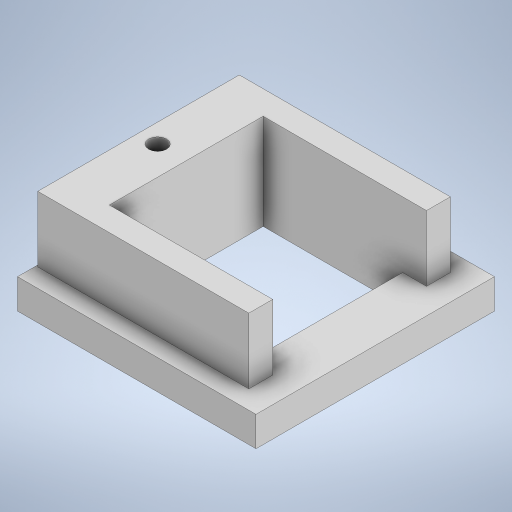
# Autodesk Inventor part: RJ45Insert
Saved by Autodesk Inventor 2024 (Build 280153000, 153)
## iProperties
Created: 2025-09-21
Part Number: RJ45Insert
Material: Generic
Document SubType Name: Modeling
Designer: Martin
Density: 1 g/cm^3
Appearance: Default
Author: Martin
Autodesk Inventor part; units mm, degrees
ref_plane "YZ Plane" through (0, 0, 0) normal (1, 0, 0) x (0, 1, 0)
ref_plane "XZ Plane" through (0, 0, 0) normal (0, 1, 0) x (-1, 0, 0)
ref_plane "XY Plane" through (0, 0, 0) normal (0, 0, 1) x (1, 0, 0)
sketch "Sketch1" plane through (0, 0, 0) normal (0, 1, 0) x (-1, 0, 0)
  line L0 (-12.7, 12.7) -> (12.7, 12.7)
  line L1 (12.7, 12.7) -> (12.7, -12.7)
  line L2 (12.7, -12.7) -> (-12.7, -12.7)
  line L3 (-12.7, -12.7) -> (-12.7, 12.7)
  line L4 (-12.7, 12.7) -> (12.7, -12.7) construction
  line L5 (12.7, 12.7) -> (-12.7, -12.7) construction
  point P0 (0, 0)
  dimension "d0" = 25.4
  dimension "d1" = 25.4
  constraints: 12 end point, 2 midpoint, 2 parallel, 1 horizontal, 1 perpendicular
  measures "d0" distance of L1.end L2.end
  measures "d1" distance of L0.end L1.end
extrude "Extrusion1" add sketch "Sketch1" along normal blind 3.175
sketch "Sketch2" plane through (0, 3.175, 0) normal (0, 1, 0) x (1, 0, 0)
  line L0 (7.4295, -8.1915) -> (-7.4295, -8.1915)
  line L1 (-7.4295, -8.1915) -> (-7.4295, 8.1915)
  line L2 (-7.4295, 8.1915) -> (7.4295, 8.1915)
  line L3 (7.4295, 8.1915) -> (7.4295, -8.1915)
  line L4 (7.4295, -8.1915) -> (-7.4295, 8.1915) construction
  line L5 (-7.4295, -8.1915) -> (7.4295, 8.1915) construction
  point P0 (0, 0)
  dimension "d4" = 14.859
  dimension "d5" = 16.383
  constraints: 12 end point, 2 midpoint, 2 parallel, 1 horizontal, 1 perpendicular
  measures "d4" distance of L1.end L2.end
  measures "d5" distance of L0.end L1.end
extrude "Extrusion2" cut sketch "Sketch2" against normal through all
sketch "Sketch3" plane through (0, 3.175, 0) normal (0, 1, 0) x (1, 0, 0)
  line L0 (-7.4295, -8.1915) -> (-7.4295, 8.1915) projected
  line L1 (-7.4295, -8.1915) -> (-12.5095, -8.1915)
  line L2 (-12.5095, -8.1915) -> (-12.5095, 8.1915)
  line L3 (-12.5095, 8.1915) -> (-7.4295, 8.1915)
  line L4 (-7.4295, 8.1915) -> (-7.4295, -8.1915)
  line L5 (-12.5095, -8.1915) -> (9.9695, -8.1915)
  line L6 (9.9695, -8.1915) -> (9.9695, -10.7315)
  line L7 (9.9695, -10.7315) -> (-12.5095, -10.7315)
  line L8 (-12.5095, -10.7315) -> (-12.5095, -8.1915)
  line L9 (7.4295, 8.1915) -> (7.4295, -8.1915) projected
  line L10 (-12.5095, 8.1915) -> (9.9695, 8.1915)
  line L11 (9.9695, 8.1915) -> (9.9695, 10.7315)
  line L12 (9.9695, 10.7315) -> (-12.5095, 10.7315)
  line L13 (-12.5095, 10.7315) -> (-12.5095, 8.1915)
  point P0 (0, 0)
  point P1 (-9.9695, 8.1915)
  point P2 (9.9695, -9.4615)
  point P3 (9.9695, 9.4615)
  dimension "d11" = 2.54
  dimension "d12" = 2.54
  dimension "d13" = 2.54
  dimension "d14" = 5.08
  constraints: 24 end point, 6 parallel, 3 horizontal, 3 midpoint, 3 perpendicular, 1 horizontal alignment, 1 vertical alignment
  measures "d11" distance of L5.end L6.end
  measures "d12" distance from line of point (9.969, -9.462) L9
  measures "d13" distance of L11.end L10.end
  measures "d14" distance between parallel lines of L2 L0
extrude "Extrusion3" add sketch "Sketch3" along normal blind 6.985 contours L1 L2 L3 L0 | L5 L6 L7 L8 L1 | L3 L13 L12 L11 L10
sketch "Sketch4" plane through (0, 10.16, 0) normal (0, 1, 0) x (1, 0, 0)
  line L0 (-7.4295, -8.1915) -> (-7.4295, 8.1915) construction
  line L1 (-7.4295, -3.81) -> (-9.7155, -3.81) construction
  line L2 (-9.7155, -3.81) -> (-9.7155, 3.81) construction
  line L3 (-9.7155, 3.81) -> (-7.4295, 3.81) construction
  line L4 (-7.4295, 3.81) -> (-7.4295, -3.81) construction
  circle A0 centre (-10.4775, 0) radius 1.143 construction
  circle A1 centre (-10.4775, 0) radius 0.9525
  point P0 (0, 0)
  point P1 (-7.4295, 0)
  point P2 (-9.7155, 0)
  dimension "d15" = 2.286
  dimension "d16" = 7.62
  dimension "d17" = 2.286
  dimension "d18" = 1.905
  dimension "d21" = 0.762
  constraints: 8 end point, 2 centre point, 2 horizontal alignment, 2 midpoint, 2 parallel, 1 coincident, 1 horizontal, 1 perpendicular, 1 point on line
  measures "d15" distance of L2.end L3.end
  measures "d16" distance of L1.end L2.end
  measures "d17" diameter of A0
  measures "d18" diameter of A1
  measures "d21" distance of point (-9.716, 0) A0.centre
extrude "Extrusion4" cut sketch "Sketch4" against normal blind 6.35
body "Solid1"
